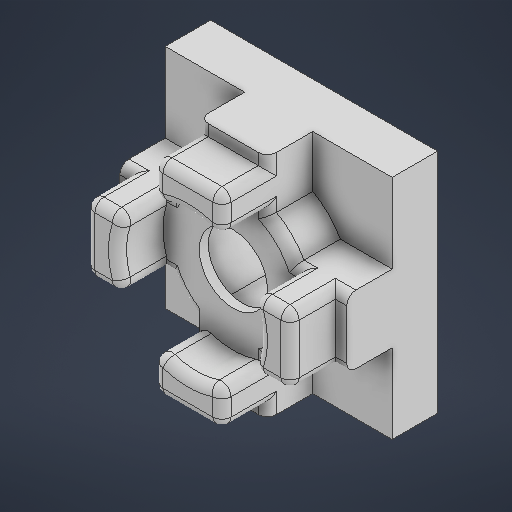
# Autodesk Inventor part: SGA
Saved by Autodesk Inventor 2026.2 (Build 302298000, 298)
## iProperties
Created: 2025-10-24
Part Number: SGA
Material: Generic
Document SubType Name: Modeling
Designer: kubek
Density: 1 g/cm^3
Appearance: Default
Author: kubek
Autodesk Inventor part; units mm, degrees
ref_plane "YZ Plane" through (0, 0, 0) normal (1, 0, 0) x (0, 1, 0)
ref_plane "XZ Plane" through (0, 0, 0) normal (0, 1, 0) x (-1, 0, 0)
ref_plane "XY Plane" through (0, 0, 0) normal (0, 0, 1) x (1, 0, 0)
sketch "Sketch1" plane through (0, 0, 0) normal (0, 0, 1) x (1, 0, 0)
  line L0 (-2.5, 2.5) -> (2.5, 2.5)
  line L1 (2.5, 2.5) -> (2.5, -2.5)
  line L2 (2.5, -2.5) -> (-2.5, -2.5)
  line L3 (-2.5, -2.5) -> (-2.5, 2.5)
  line L4 (-2.5, 2.5) -> (2.5, -2.5) construction
  line L5 (2.5, 2.5) -> (-2.5, -2.5) construction
  point P0 (0, 0)
  dimension "d0" = 5
  dimension "d1" = 5
  constraints: 12 end point, 2 midpoint, 2 parallel, 1 horizontal, 1 perpendicular
  measures "d0" distance of L1.end L2.end
  measures "d1" distance of L0.end L1.end
extrude "Extrusion1" add sketch "Sketch1" along normal blind 2
sketch "Sketch10" plane through (0, 0, 2) normal (0, 0, 1) x (1, 0, 0)
  circle A0 centre (0, 0) radius 0.75
  dimension "d145" = 1.5
  constraints: 1 centre point, 1 coincident
  measures "d145" diameter of A0
extrude "Extrusion8" cut sketch "Sketch10" against normal blind 10
sketch "Sketch11" plane through (0, 0, 0) normal (0, 0, -1) x (-1, 0, 0)
  circle A0 centre (0, 0) radius 1.1
  line L0 (0.635085, 1.1) -> (1.270171, 0)
  line L1 (1.270171, 0) -> (0.635085, -1.1)
  line L2 (0.635085, -1.1) -> (-0.635085, -1.1)
  line L3 (-0.635085, -1.1) -> (-1.270171, 0)
  line L4 (-1.270171, 0) -> (-0.635085, 1.1)
  line L5 (-0.635085, 1.1) -> (0.635085, 1.1)
  point P0 (0, 1.1)
  point P1 (-0.952628, 0.55)
  point P2 (0.952628, 0.55)
  point P3 (-0.952628, -0.55)
  point P4 (0, -1.1)
  point P5 (0.952628, -0.55)
  dimension "d148" = 2.2
  constraints: 12 end point, 2 coincident, 1 midpoint, 16 other
extrude "Extrusion9" cut sketch "Sketch11" against normal blind 1.8
sketch "Sketch12" plane through (0, 0, 2) normal (0, 0, 1) x (1, 0, 0)
  circle A0 centre (0, 0) radius 1.3
  line L0 (2.5, 2.5) -> (-2.5, 2.5)
  line L1 (-2.5, -2.5) -> (2.5, -2.5)
  line L2 (-2.5, 2.5) -> (2.5, 2.5)
  line L3 (2.5, 2.5) -> (2.5, -2.5)
  line L4 (2.5, -2.5) -> (-2.5, -2.5)
  line L5 (-2.5, -2.5) -> (-2.5, 2.5)
  line L6 (-2.25, 2.25) -> (2.25, 2.25)
  line L7 (2.25, 2.25) -> (2.25, -2.25)
  line L8 (2.25, -2.25) -> (-2.25, -2.25)
  line L9 (-2.25, -2.25) -> (-2.25, 2.25)
  line L10 (2.5, -2.5) -> (2.5, 2.5)
  line L11 (-2.5, 2.5) -> (-2.5, -2.5)
  arc A1 (-1, -1.184272) -> (1, -1.184272) centre (0, 0) ccw
  circle A2 centre (0, 0) radius 1.55
  line L12 (-1, 2.25) -> (-1, 0.830662)
  line L13 (-0.75, 2.5) -> (-0.75, 1.061838)
  line L14 (0.75, 2.5) -> (0.75, 1.061838)
  line L15 (1, 2.5) -> (1, 0.830662)
  line L16 (-0.75, -2.25) -> (-0.75, -1.061838)
  line L17 (-1, -2.25) -> (-1, -0.830662)
  line L18 (0.75, -2.25) -> (0.75, -1.061838)
  line L19 (1, -2.25) -> (1, -0.830662)
  line L20 (-2.25, 1) -> (-0.830662, 1)
  line L21 (-2.25, 0.75) -> (-1.061838, 0.75)
  line L22 (-2.25, -0.75) -> (-1.061838, -0.75)
  line L23 (-2.25, -1) -> (-0.830662, -1)
  line L24 (0.830662, 1) -> (2.25, 1)
  line L25 (1.061838, 0.75) -> (2.25, 0.75)
  line L26 (0.830662, -1) -> (2.25, -1)
  line L27 (1.061838, -0.75) -> (2.25, -0.75)
  line L28 (-2.25, 1) -> (-2.5, 1)
  line L29 (-2.25, 0.75) -> (-2.5, 0.75)
  line L30 (-2.25, -0.75) -> (-2.5, -0.75)
  line L31 (-2.25, -1) -> (-2.5, -1)
  line L32 (-1, -2.25) -> (-1, -2.5)
  line L33 (-0.75, -2.25) -> (-0.75, -2.5)
  line L34 (0.75, -2.25) -> (0.75, -2.5)
  line L35 (1, -2.25) -> (1, -2.5)
  line L36 (2.25, -1) -> (2.5, -1)
  line L37 (2.25, -0.75) -> (2.5, -0.75)
  line L38 (2.25, 0.75) -> (2.5, 0.75)
  line L39 (2.25, 1) -> (2.5, 1)
  line L40 (-1, 2.25) -> (-1, 2.5)
  point P0 (0.75, 1.780919)
  point P1 (1.356466, -0.75)
  point P2 (1.356466, 0.75)
  point P3 (0.75, -1.356466)
  point P4 (-0.75, -1.356466)
  point P5 (-1.356466, -0.75)
  point P6 (-1.356466, 0.75)
  point P7 (0.75, 1.356466)
  point P8 (0.75, 2.25)
  point P9 (-0.75, 2.25)
  point P10 (-0.75, 1.356466)
  point P11 (-1, -1.184272)
  point P12 (1, -1.184272)
  dimension "d151" = 2.6
  dimension "d153" = 0.25
  dimension "d154" = 0.25
  dimension "d155" = 0.25
  dimension "d156" = 0.25
  dimension "d167" = 5
  dimension "d168" = 5
  dimension "d181" = 1.25
  dimension "d182" = 0.25
  dimension "d183" = 1.5
  dimension "d184" = 0.25
  dimension "d185" = 1.25
  dimension "d186" = 1.25
  dimension "d187" = 0.25
  dimension "d188" = 1.5
  dimension "d189" = 0.25
  dimension "d190" = 1.25
  dimension "d191" = 0.25
  dimension "d192" = 1.5
  dimension "d193" = 0.25
  dimension "d194" = 1.25
  constraints: 74 end point, 36 point on line, 14 perpendicular, 10 parallel, 5 horizontal, 3 coincident, 2 centre point, 2 point on circle, 2 vertical, 1 midpoint, 18 other
  measures "d153" distance between parallel lines of L5 L9
  measures "d154" distance between parallel lines of L0 L6
  measures "d155" distance between parallel lines of L1 L8
  measures "d156" distance between parallel lines of L3 L7
  measures "d167" distance of L4.end L0.end
  measures "d168" distance of L0.start L0.end
  measures "d181" distance between parallel lines of L9 L12
  measures "d182" distance between parallel lines of L12 L13
  measures "d183" distance from line of point (0.75, 1.781) L13
  measures "d184" distance between parallel lines of L15 L14
  measures "d185" distance between parallel lines of L7 L15
  measures "d186" distance between parallel lines of L6 L20
  measures "d187" distance between parallel lines of L21 L20
  measures "d188" distance between parallel lines of L22 L21
  measures "d189" distance between parallel lines of L23 L22
  measures "d190" distance between parallel lines of L24 L6
  measures "d191" distance between parallel lines of L25 L24
  measures "d192" distance between parallel lines of L27 L25
  measures "d193" distance between parallel lines of L26 L27
  measures "d194" distance between parallel lines of L8 L26
extrude "Extrusion10" add sketch "Sketch12" along normal blind 1 contours L25 L7 L27 A2 | A2 L13 L6 L14 | L18 L8 L16 A1 | A2 L22 L9 L21
extrude "Extrusion11" cut sketch "Sketch12" against normal blind 1 contours A2 L24 L7 L25 | L27 L7 L26 A2 | A2 L15 L6 L7 L24 | L7 L39 L3 L38 | L26 L7 L8 L19 A2 | L37 L3 L36 L7 | A2 L14 L6 L15 | L7 L6 L15 L0 L3 L39 | L19 L8 L18 A1 | L36 L3 L1 L35 L8 L7 | L6 L14 L0 L15 | L35 L1 L34 L8 | A2 L12 L6 L13 | L16 L8 L17 A1 | A2 L20 L9 L6 L12 | L6 L40 L0 L13 | L17 L8 L9 L23 A2 | L33 L1 L32 L8 | A2 L21 L9 L20 | L6 L9 L28 L5 L0 L40 | L23 L9 L22 A2 | L32 L1 L5 L31 L9 L8 | L9 L29 L5 L28 | L31 L5 L30 L9
fillet "Fillet1" radius 0.2 44 edges at (-1.096, -1.096, 2) (-2.375, 0.75, 2) (-0.75, -2.375, 2) (0, -1.55, 3) (-0.75, -1.3565, 2.5) (-0.75, -1.8032, 3) (-0.75, -2.25, 2.5) (0, -2.25, 3) (-1.55, 0, 3) (-1.8032, 0.75, 3) (-2.25, 0, 3) (-1.8032, -0.75, 3) (1.55, 0, 3) (1.3565, -0.75, 2.5) (-1.3565, 0.75, 2.5) (-2.25, 0.75, 2.5) (-2.25, -0.75, 2.5) (-1.3565, -0.75, 2.5) (-1.096, 1.096, 2) (-0.75, 2.375, 2) (0, 2.25, 3) (-0.75, 1.8032, 3) (0, 1.55, 3) (0.75, 1.8032, 3) (-0.75, 2.25, 2.5) (-0.75, 1.3565, 2.5) (0.75, 1.3565, 2.5) (0.75, 2.25, 2.5) (2.25, 0, 3) (1.8032, -0.75, 3) (2.25, -0.75, 2.5) (0.75, 2.375, 2) (2.25, 0.75, 2.5) (1.8032, 0.75, 3) (1.3565, 0.75, 2.5) (2.375, 0.75, 2) (1.096, 1.096, 2) (-2.375, -0.75, 2) (1.096, -1.096, 2) (0.75, -2.25, 2.5) (0.75, -1.8032, 3) (0.75, -1.3565, 2.5) (0.75, -2.375, 2) (2.375, -0.75, 2)
fillet "Fillet2" radius 0.2 12 edges at (-1.5089, -0.75, 2) (-1.2395, -0.75, 2) (-1.5089, 0.75, 2) (-1.2395, 0.75, 2) (0.75, 1.5089, 2) (0.75, 1.2395, 2) (1.5089, 0.75, 2) (1.2395, 0.75, 2) (1.5089, -0.75, 2) (1.2395, -0.75, 2) (0.75, -1.5089, 2) (0.75, -1.2395, 2)
body "Solid1"
